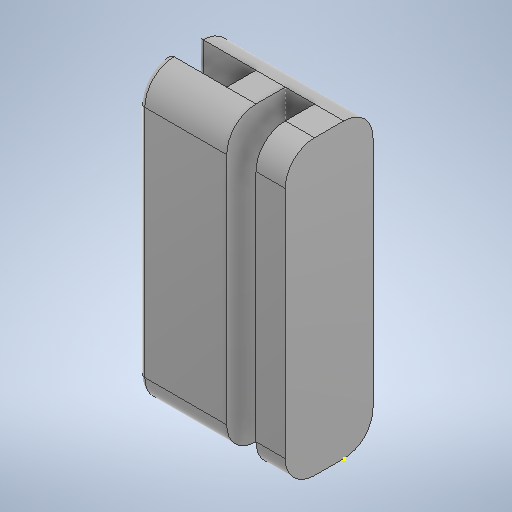
# Autodesk Inventor part: TSU_Middle_Clamp
Saved by Autodesk Inventor 2025.2 (Build 292293000, 293)
## iProperties
Created: 2025-01-07
Part Number: TSU_Middle_Clamp
Material: Generic
Document SubType Name: Modeling
Designer: Matt Tidd
Density: 1 g/cm^3
Appearance: Default
Author: Matt Tidd
Autodesk Inventor part; units mm, degrees
ref_plane "YZ Plane" through (0, 0, 0) normal (1, 0, 0) x (0, 1, 0)
ref_plane "XZ Plane" through (0, 0, 0) normal (0, 1, 0) x (-1, 0, 0)
ref_plane "XY Plane" through (0, 0, 0) normal (0, 0, 1) x (1, 0, 0)
sketch "Sketch1" plane through (0, 0, 0) normal (0, 1, 0) x (-1, 0, 0)
  line L0 (0, 0) -> (10, 0)
  line L1 (10, 0) -> (10, -20)
  line L2 (10, -20) -> (0, -20)
  line L3 (0, -20) -> (0, 0)
  line L4 (20, 0) -> (30, 0)
  line L5 (30, 0) -> (30, -20)
  line L6 (30, -20) -> (20, -20)
  line L7 (20, -20) -> (20, 0)
  line L8 (30, -20) -> (0, -20)
  line L9 (0, -20) -> (0, -30)
  line L10 (0, -30) -> (30, -30)
  line L11 (30, -30) -> (30, -20)
  dimension "d7" = 10
  dimension "d8" = 20
  dimension "d9" = 10
  dimension "d10" = 10
  constraints: 24 end point, 6 parallel, 3 horizontal, 3 perpendicular
  measures "d7" distance of L1.end L2.end
  measures "d8" distance of L0.end L1.end
  measures "d9" distance of L5.end L6.end
  measures "d10" distance of L9.end L8.end
extrude "Extrusion1" add sketch "Sketch1" along normal blind 100
sketch "Sketch2" plane through (-30, 0, -30) normal (-1, 0, 0) x (0, 0, 1)
  line L0 (30, 0) -> (0, 0) projected
  line L1 (0, 0) -> (10, 0)
  line L2 (10, 0) -> (10, 100)
  line L3 (10, 100) -> (0, 100)
  line L4 (0, 100) -> (0, 0)
  line L5 (30, 0) -> (30, 100) projected
  line L6 (30, 100) -> (20, 100)
  line L7 (20, 100) -> (20, 0)
  line L8 (20, 0) -> (30, 0)
  line L9 (30, 0) -> (30, 100)
  dimension "d11" = 10
  dimension "d12" = 100
  dimension "d13" = 10
  constraints: 16 end point, 4 parallel, 2 horizontal, 2 perpendicular, 1 point on line
  measures "d11" distance of L3.end L2.end
  measures "d12" distance of L2.end L1.end
  measures "d13" distance of L8.end L7.end
extrude "Extrusion2" add sketch "Sketch2" along normal blind 20
sketch "Sketch3" plane through (-20, 0, -20) normal (0, 0, 1) x (1, 0, 0)
  line L0 (0, 0) -> (0, 100) construction
  line L1 (0, 50) -> (10, 50) construction
  line L2 (10, 0) -> (10, 100) construction
  point P0 (20, 0)
  constraints: 2 end point, 2 midpoint
fillet "Fillet1" radius 10 6 edges at (-35, 100, 0) (-5, 100, 0) (-5, 0, 0) (-35, 0, 0) (-25, 0, -30) (-25, 100, -30)
fillet "Fillet2" radius 2 12 edges at (-50, 0, -20.0001) (-50, 2.9289, -27.0711) (-50, 97.0711, -27.0711) (-50, 100, -20.0001) (-50, 50, -30) (-50, 50, -20) (-50, 0, -9.9999) (-50, 100, -9.9999) (-50, 50, -10) (-50, 97.0711, -2.9289) (-50, 2.9289, -2.9289) (-50, 50, 0)
body "Solid1"
